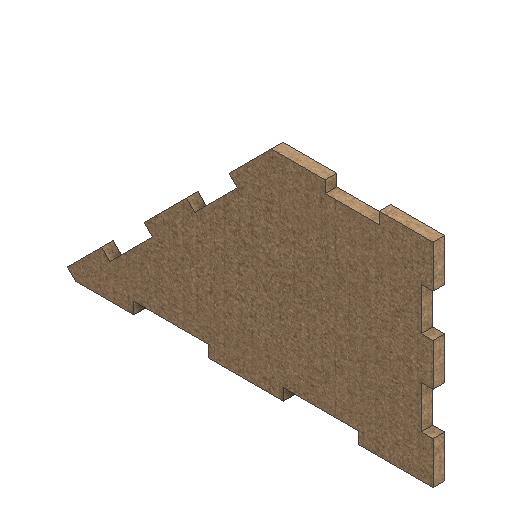
# Autodesk Inventor part: SidePlate
Saved by Autodesk Inventor 2025.2 (Build 292293000, 293)
## iProperties
Created: 2025-03-07
Part Number: SidePlate
Material: MDF Medium Density Fiberboard
Document SubType Name: Modeling
Designer: ahorat
Density: 0.8 g/cm^3
Appearance: Cardboard - Corrugated
Author: ahorat
Autodesk Inventor part; units mm, degrees
ref_plane "YZ Plane" through (0, 0, 0) normal (1, 0, 0) x (0, 1, 0)
ref_plane "XZ Plane" through (0, 0, 0) normal (0, 1, 0) x (-1, 0, 0)
ref_plane "XY Plane" through (0, 0, 0) normal (0, 0, 1) x (1, 0, 0)
sketch "Sketch1" plane through (0, 0, 0) normal (0, 0, 1) x (1, 0, 0)
  line L0 (0, 0) -> (0, 92)
  line L1 (0, 92) -> (-70, 92)
  line L2 (-70, 92) -> (-161.8477, 0)
  line L3 (-161.8477, 0) -> (0, 0)
  dimension "d1" = 70
  dimension "d2" = 130
  dimension "d7" = 92
  constraints: 8 end point, 1 parallel, 1 perpendicular, 1 vertical
  measures "d1" distance of L0.end L1.end
  measures "d2" distance of L1.end L2.end
  measures "d7" distance of L0.start L0.end
extrude "Extrusion1" add sketch "Sketch1" along normal blind 5
sketch "Sketch2" plane through (0, 0, 5) normal (0, 0, 1) x (1, 0, 0)
  line L0 (-70, 92) -> (-161.8477, 0) projected
  line L1 (-143.5135, 18.3646) -> (-139.9043, 14.7614)
  line L2 (-139.9043, 14.7614) -> (-121.4641, 33.2321)
  line L3 (-121.4641, 33.2321) -> (-125.0733, 36.8354)
  line L4 (-106.7744, 55.1646) -> (-103.1652, 51.5614)
  line L5 (-103.1652, 51.5614) -> (-84.725, 70.0321)
  line L6 (-84.725, 70.0321) -> (-88.3342, 73.6354)
  line L7 (-123.2687, 35.0338) -> (-104.9698, 53.363) construction
  line L8 (-114.1192, 44.1984) -> (-115.9239, 46)
  line L9 (-161.8477, 0) -> (0, 0) projected
  line L10 (-129.5282, 0) -> (-97.0586, 0)
  line L11 (-97.0586, 0) -> (-97.0586, 5.1)
  line L12 (-97.0586, 5.1) -> (-129.5282, 5.1)
  line L13 (-129.5282, 5.1) -> (-129.5282, 0)
  line L14 (-64.7891, 0) -> (-32.3195, 0)
  line L15 (-32.3195, 0) -> (-32.3195, 5.1)
  line L16 (-32.3195, 5.1) -> (-64.7891, 5.1)
  line L17 (-64.7891, 5.1) -> (-64.7891, 0)
  line L18 (0, 18.35) -> (-5.1, 18.35)
  line L19 (-5.1, 18.35) -> (-5.1, 36.85)
  line L20 (-5.1, 36.85) -> (0, 36.85)
  line L21 (0, 36.85) -> (0, 18.35)
  line L22 (0, 55.15) -> (-5.1, 55.15)
  line L23 (-5.1, 55.15) -> (-5.1, 73.65)
  line L24 (-5.1, 73.65) -> (0, 73.65)
  line L25 (0, 73.65) -> (0, 55.15)
  line L26 (0, 92) -> (-70, 92) projected
  line L27 (-46.7167, 92) -> (-23.2833, 92)
  line L28 (-23.2833, 92) -> (-23.2833, 86.9)
  line L29 (-23.2833, 86.9) -> (-46.7167, 86.9)
  line L30 (-46.7167, 86.9) -> (-46.7167, 92)
  line L31 (0, 0) -> (0, 92) projected
  line L32 (-2.55, 36.85) -> (-2.55, 55.15) construction
  line L33 (-64.7891, 2.55) -> (-97.0586, 2.55) construction
  point P0 (-35, 86.9)
  point P1 (-35, 92)
  point P2 (-80.9239, 2.55)
  point P3 (-80.9239, 0)
  point P4 (-2.55, 46)
  point P5 (0, 46)
  point P6 (-35, 92)
  dimension "d8" = 130
  dimension "d9" = 26.1
  dimension "d10" = 25.9
  dimension "d13" = 5.1
  dimension "d14" = 70
  dimension "d15" = 92
  dimension "d16" = 161.8477
  dimension "d17" = 32.2695
  dimension "d18" = 32.4695
  dimension "d19" = 18.3
  dimension "d20" = 18.5
  dimension "d21" = 23.4333
  constraints: 60 end point, 15 midpoint, 12 point on line, 11 perpendicular, 10 parallel, 6 equal length, 6 horizontal, 3 vertical alignment, 1 horizontal alignment, 1 vertical
  measures "d8" distance of L0.start L0.end
  measures "d9" distance of L4.end L5.end
  measures "d10" distance of L7.start L7.end
  measures "d13" distance of L5.end L6.end
  measures "d14" distance of L26.start L0.start
  measures "d15" distance between parallel lines of L9 L26
  measures "d16" distance from line of L0.end L31
  measures "d17" distance of L33.start L33.end
  measures "d18" distance of L11.end L12.end
  measures "d19" distance of L32.start L32.end
  measures "d20" distance of L18.end L19.end
  measures "d21" distance of L28.end L29.end
extrude "Extrusion2" cut sketch "Sketch2" against normal blind 10 contours L6 L5 L4 L0 | L26 L28 L29 L30 | L3 L2 L1 L0 | L25 L22 L23 L24 | L21 L18 L19 L20 | L13 L12 L11 L9 | L17 L16 L15 L9
sketch "Sketch3" plane through (0, 0, 5) normal (0, 0, 1) x (1, 0, 0)
  line L0 (-5.1, 36.85) -> (0, 36.85) projected
  line L1 (0, 36.85) -> (0, 55.15) projected
  line L2 (0, 55.15) -> (-5.1, 55.15) projected
  line L3 (-5.1, 55.15) -> (-5.1, 73.65) projected
  line L4 (-5.1, 73.65) -> (0, 73.65) projected
  line L5 (0, 73.65) -> (0, 92) projected
  line L6 (0, 92) -> (-23.2833, 92) projected
  line L7 (-23.2833, 92) -> (-23.2833, 86.9) projected
  line L8 (-23.2833, 86.9) -> (-46.7167, 86.9) projected
  line L9 (-46.7167, 86.9) -> (-46.7167, 92) projected
  line L10 (-46.7167, 92) -> (-70, 92) projected
  line L11 (-70, 92) -> (-88.3342, 73.6354) projected
  line L12 (-88.3342, 73.6354) -> (-84.725, 70.0321) projected
  line L13 (-84.725, 70.0321) -> (-103.1652, 51.5614) projected
  line L14 (-103.1652, 51.5614) -> (-106.7744, 55.1646) projected
  line L15 (-106.7744, 55.1646) -> (-125.0733, 36.8354) projected
  line L16 (-125.0733, 36.8354) -> (-121.4641, 33.2321) projected
  line L17 (-121.4641, 33.2321) -> (-139.9043, 14.7614) projected
  line L18 (-139.9043, 14.7614) -> (-143.5135, 18.3646) projected
  line L19 (-143.5135, 18.3646) -> (-161.8477, 0) projected
  line L20 (-161.8477, 0) -> (-129.5282, 0) projected
  line L21 (-129.5282, 0) -> (-129.5282, 5.1) projected
  line L22 (-129.5282, 5.1) -> (-97.0586, 5.1) projected
  line L23 (-97.0586, 5.1) -> (-97.0586, 0) projected
  line L24 (-97.0586, 0) -> (-64.7891, 0) projected
  line L25 (-64.7891, 0) -> (-64.7891, 5.1) projected
  line L26 (-64.7891, 5.1) -> (-32.3195, 5.1) projected
  line L27 (-32.3195, 5.1) -> (-32.3195, 0) projected
  line L28 (-32.3195, 0) -> (0, 0) projected
  line L29 (0, 0) -> (0, 18.35) projected
  line L30 (0, 18.35) -> (-5.1, 18.35) projected
  line L31 (-5.1, 18.35) -> (-5.1, 36.85) projected
  line L32 (-132.1444, 36.8295) -> (-106.7803, 62.2357)
  line L33 (-106.7803, 62.2357) -> (-103.171, 58.6324)
  line L34 (-103.171, 58.6324) -> (-91.796, 70.0263)
  line L35 (-91.796, 70.0263) -> (-95.4053, 73.6295)
  line L36 (-95.4053, 73.6295) -> (-72.0735, 97)
  line L37 (-72.0735, 97) -> (-41.7167, 97)
  line L38 (-41.7167, 97) -> (-41.7167, 91.9)
  line L39 (-41.7167, 91.9) -> (-28.2833, 91.9)
  line L40 (-28.2833, 91.9) -> (-28.2833, 97)
  line L41 (-28.2833, 97) -> (5, 97)
  line L42 (5, 97) -> (5, 68.65)
  line L43 (5, 68.65) -> (-0.1, 68.65)
  line L44 (-0.1, 68.65) -> (-0.1, 60.15)
  line L45 (-0.1, 60.15) -> (5, 60.15)
  line L46 (5, 60.15) -> (5, 31.85)
  line L47 (5, 31.85) -> (-0.1, 31.85)
  line L48 (-0.1, 31.85) -> (-0.1, 23.35)
  line L49 (-0.1, 23.35) -> (5, 23.35)
  line L50 (5, 23.35) -> (5, -5)
  line L51 (5, -5) -> (-37.3195, -5)
  line L52 (-37.3195, -5) -> (-37.3195, 0.1)
  line L53 (-37.3195, 0.1) -> (-59.7891, 0.1)
  line L54 (-59.7891, 0.1) -> (-59.7891, -5)
  line L55 (-59.7891, -5) -> (-102.0586, -5)
  line L56 (-102.0586, -5) -> (-102.0586, 0.1)
  line L57 (-102.0586, 0.1) -> (-124.5282, 0.1)
  line L58 (-124.5282, 0.1) -> (-124.5282, -5)
  line L59 (-124.5282, -5) -> (-173.9046, -5)
  line L60 (-173.9046, -5) -> (-143.5193, 25.4357)
  line L61 (-143.5193, 25.4357) -> (-139.9101, 21.8324)
  line L62 (-139.9101, 21.8324) -> (-128.5351, 33.2263)
  line L63 (-128.5351, 33.2263) -> (-132.1444, 36.8295)
  line L64 (-143.5135, 18.3646) -> (-147.0519, 21.8972)
  line L65 (-161.8477, 0) -> (-168.9129, 0)
  line L66 (-125.0733, 36.8354) -> (-128.6118, 40.368)
  line L67 (-106.7744, 55.1646) -> (-110.3129, 58.6972)
  line L68 (-103.171, 58.6324) -> (-106.7744, 55.1646)
  line L69 (-91.796, 70.0263) -> (-88.3342, 73.6354)
  line L70 (-88.3342, 73.6354) -> (-91.8727, 77.168)
  line L71 (-70, 92) -> (-77.0652, 92)
  line L72 (-139.9101, 21.8324) -> (-143.5135, 18.3646)
  line L73 (-125.0733, 36.8354) -> (-128.5351, 33.2263)
  line L74 (-143.5135, 18.3646) -> (-161.8477, 0) projected
  line L75 (-161.8477, 0) -> (-165.3862, 3.5326)
  dimension "d22" = 5
  constraints: 86 end point, 8 point on line, 4 perpendicular, 1 horizontal, 1 parallel, 31 other
  measures "d22" distance between parallel lines of L15 L32
extrude "Extrusion3" [suppressed]
sketch "Sketch4" plane through (0, 0, 5) normal (0, 0, 1) x (1, 0, 0)
  line L0 (-5.1, 36.85) -> (0, 36.85) projected
  line L1 (0, 36.85) -> (0, 55.15) projected
  line L2 (0, 55.15) -> (-5.1, 55.15) projected
  line L3 (-5.1, 55.15) -> (-5.1, 73.65) projected
  line L4 (-5.1, 73.65) -> (0, 73.65) projected
  line L5 (0, 73.65) -> (0, 92) projected
  line L6 (0, 92) -> (-23.2833, 92) projected
  line L7 (-23.2833, 92) -> (-23.2833, 86.9) projected
  line L8 (-23.2833, 86.9) -> (-46.7167, 86.9) projected
  line L9 (-46.7167, 86.9) -> (-46.7167, 92) projected
  line L10 (-46.7167, 92) -> (-70, 92) projected
  line L11 (-70, 92) -> (-88.3342, 73.6354) projected
  line L12 (-88.3342, 73.6354) -> (-84.725, 70.0321) projected
  line L13 (-84.725, 70.0321) -> (-103.1652, 51.5614) projected
  line L14 (-103.1652, 51.5614) -> (-106.7744, 55.1646) projected
  line L15 (-106.7744, 55.1646) -> (-125.0733, 36.8354) projected
  line L16 (-125.0733, 36.8354) -> (-121.4641, 33.2321) projected
  line L17 (-121.4641, 33.2321) -> (-139.9043, 14.7614) projected
  line L18 (-139.9043, 14.7614) -> (-143.5135, 18.3646) projected
  line L19 (-143.5135, 18.3646) -> (-161.8477, 0) projected
  line L20 (-161.8477, 0) -> (-129.5282, 0) projected
  line L21 (-129.5282, 0) -> (-129.5282, 5.1) projected
  line L22 (-129.5282, 5.1) -> (-97.0586, 5.1) projected
  line L23 (-97.0586, 5.1) -> (-97.0586, 0) projected
  line L24 (-97.0586, 0) -> (-64.7891, 0) projected
  line L25 (-64.7891, 0) -> (-64.7891, 5.1) projected
  line L26 (-64.7891, 5.1) -> (-32.3195, 5.1) projected
  line L27 (-32.3195, 5.1) -> (-32.3195, 0) projected
  line L28 (-32.3195, 0) -> (0, 0) projected
  line L29 (0, 0) -> (0, 18.35) projected
  line L30 (0, 18.35) -> (-5.1, 18.35) projected
  line L31 (-5.1, 18.35) -> (-5.1, 36.85) projected
  line L32 (-143.5135, 18.3646) -> (-161.8477, 0) projected
  line L33 (-158.3209, 3.5326) -> (-154.7825, 0)
  dimension "d27" = 5
  constraints: 2 end point, 2 point on line, 1 perpendicular
  measures "d27" distance of L33.start L33.end
extrude "Extrusion4" cut sketch "Sketch4" against normal through all contours L20 L19 L33
body "Solid1"
